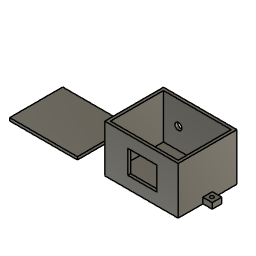
Box and lid v1 (Autodesk Fusion 360 design; units mm, degrees)
Autodesk Fusion 360 part; units mm, degrees
sketch "Sketch4" plane through (0, 0, 0) normal (0, 0, 1) x (1, 0, 0)
  line L0 (38.75, -31) -> (-38.75, -31)
  line L1 (-38.75, -31) -> (-38.75, 31)
  line L2 (-38.75, 31) -> (38.75, 31)
  line L3 (38.75, 31) -> (38.75, -31)
  line L4 (38.75, -31) -> (-38.75, 31) construction
  line L5 (-38.75, -31) -> (38.75, 31) construction
  dimension "d14" = 77.5
  dimension "d15" = 62
  constraint horizontal L0
  constraint perpendicular L0 L1
  constraint parallel L0 L2
  constraint parallel L1 L3
  constraint coincident L4 origin
  constraint coincident L5 origin
  measures "d14" distance of L1 L3
  measures "d15" distance of L0 L2
extrude "Extrude4" add sketch "Sketch4" along normal blind 50 makes body 1
sketch "Sketch5" plane through (0, 0, 50) normal (0, 0, 1) x (-1, 0, 0)
  line L0 (-38.75, -31) -> (38.75, -31)
  line L1 (38.75, -31) -> (38.75, 31)
  line L2 (38.75, 31) -> (-38.75, 31)
  line L3 (-38.75, 31) -> (-38.75, -31)
  line L4 (-35.75, 28) -> (35.75, 28)
  line L5 (35.75, 28) -> (35.75, -28)
  line L6 (35.75, -28) -> (-35.75, -28)
  line L7 (-35.75, -28) -> (-35.75, 28)
  line L8 (-35.75, 28) -> (35.75, -28) construction
  line L9 (35.75, 28) -> (-35.75, -28) construction
  dimension "d18" = 71.5
  dimension "d19" = 56
  constraint horizontal L4
  constraint perpendicular L4 L5
  constraint parallel L4 L6
  constraint parallel L5 L7
  constraint coincident L8 origin
  constraint coincident L9 origin
  measures "d18" distance of L5 L7
  measures "d19" distance of L4 L6
extrude "Extrude5" cut sketch "Sketch5" against normal blind 47 contours L4 L5 L6 L7 bodies 1
sketch "Sketch6" plane through (0, -31, 0) normal (0, -1, 0) x (1, 0, 0)
  line L0 (-38.75, 0) -> (38.75, 0)
  line L1 (38.75, 0) -> (38.75, 50)
  line L2 (38.75, 50) -> (-38.75, 50)
  line L3 (-38.75, 50) -> (-38.75, 0)
  line L4 (16.143, 12.6054) -> (-14.457, 12.6054)
  line L5 (-14.457, 12.6054) -> (-14.457, 37.3554)
  line L6 (-14.457, 37.3554) -> (16.143, 37.3554)
  line L7 (16.143, 37.3554) -> (16.143, 12.6054)
  line L8 (16.143, 12.6054) -> (-14.457, 37.3554) construction
  line L9 (-14.457, 12.6054) -> (16.143, 37.3554) construction
  point P0 (0.843, 24.9804)
  dimension "d22" = 30.6
  dimension "d23" = 24.75
  constraint horizontal L4
  constraint perpendicular L4 L5
  constraint parallel L4 L6
  constraint parallel L5 L7
  constraint coincident L8 P0
  constraint coincident L9 P0
  measures "d22" distance of L5 L7
  measures "d23" distance of L4 L6
extrude "Extrude6" cut sketch "Sketch6" against normal blind 5 contours L4 L5 L6 L7 bodies 1
sketch "Sketch7" plane through (0, 31, 0) normal (0, 1, 0) x (-1, 0, 0)
  line L0 (-38.75, 0) -> (38.75, 0)
  line L1 (38.75, 0) -> (38.75, 50)
  line L2 (38.75, 50) -> (-38.75, 50)
  line L3 (-38.75, 50) -> (-38.75, 0)
  line L4 (0, 60) -> (0, -15)
  circle A0 centre (-20, 25) radius 3.675
  circle A1 centre (20, 25) radius 3.675
  dimension "d26" = 7.35
  dimension "d27" = 7.35
  constraint perpendicular L0 L4
  measures "d26" diameter of A0
  measures "d27" diameter of A1
extrude "Extrude7" cut sketch "Sketch7" against normal blind 5 contours A0 bodies 1
extrude "Extrude8" cut sketch "Sketch7" against normal blind 5 contours A1 bodies 1
sketch "Sketch8" plane through (0, 0, 3) normal (0, 0, 1) x (-1, 0, 0)
  line L0 (-35.75, -28) -> (35.75, -28)
  line L1 (35.75, -28) -> (35.75, 28)
  line L2 (35.75, 28) -> (-35.75, 28)
  line L3 (-35.75, 28) -> (-35.75, -28)
  line L4 (49, -5) -> (39, -5)
  line L5 (39, -5) -> (39, 5)
  line L6 (39, 5) -> (49, 5)
  line L7 (49, 5) -> (49, -5)
  dimension "d32" = 10
  dimension "d33" = 10
  constraint horizontal L4
  constraint vertical L5
  constraint horizontal L6
  constraint vertical L7
  measures "d32" distance of L5 L7
  measures "d33" distance of L4 L6
extrude "Extrude9" add sketch "Sketch8" along normal blind 6 separate body contours L4 L5 L6 L7 makes body 2
move_body "Move1" bodies 2 to x (1, 0, 0) y (0, 1, 0) z (0, 0, 1) at (0, 0, -3)
sketch "Sketch9" plane through (0, 0, 3) normal (0, 0, 1) x (1, 0, 0)
move_body "Move2" bodies 2 to x (1, 0, 0) y (0, 1, 0) z (0, 0, 1) at (0.2552, 0.0123, 0.0295)
copy_body "CopyPasteBodies1" bodies 2 makes body 3
move_body "Move3" bodies 3 to x (1, 0, 0) y (0, -1, 0) z (0, 0, -1) at (87.4885, 0.0371, 6.207)
sketch "Sketch10" plane through (0, 0, 6.0295) normal (0, 0, 1) x (-1, 0, 0)
  line L0 (48.7448, 4.9877) -> (38.7448, 4.9877)
  line L1 (38.7448, 4.9877) -> (38.7448, -5.0123)
  line L2 (38.7448, -5.0123) -> (48.7448, -5.0123)
  line L3 (48.7448, -5.0123) -> (48.7448, 4.9877)
  circle A0 centre (43.5, 0) radius 1.825
  circle A1 centre (43.5, 0) radius 1.825
  point P0 (-43.5043, -0.185)
  point P1 (43.5, 0)
  dimension "d36" = 3.65
  dimension "d37" = 3.65
  constraint coincident P1 A0.centre
  measures "d36" diameter of A0
  measures "d37" diameter of A1
extrude "Extrude10" cut sketch "Sketch10" against normal blind 6 contours A0 A1 bodies 2
sketch "Sketch11" plane through (0, 0, 6.1775) normal (0, 0, 1) x (-1, 0, 0)
  line L0 (-48.7437, -5.0248) -> (-38.7437, -5.0248)
  line L1 (-38.7437, -5.0248) -> (-38.7437, 4.9752)
  line L2 (-38.7437, 4.9752) -> (-48.7437, 4.9752)
  line L3 (-48.7437, 4.9752) -> (-48.7437, -5.0248)
  circle A0 centre (-43.4472, -0.0093) radius 1.825
  dimension "d40" = 3.65
  measures "d40" diameter of A0
extrude "Extrude11" cut sketch "Sketch11" against normal blind 6 contours A0 bodies 3
combine "Combine1" operation add target body 2 tool bodies 1 3
sketch "Sketch13" plane through (0, 0, 50) normal (0, 0, 1) x (-1, 0, 0)
  line L0 (35.75, 28) -> (35.75, -28)
  line L1 (35.75, -28) -> (-35.75, -28)
  line L2 (-35.75, -28) -> (-35.75, 28)
  line L3 (-35.75, 28) -> (35.75, 28)
  line L4 (-38.75, -31) -> (38.75, -31)
  line L5 (38.75, -31) -> (38.75, 31)
  line L6 (38.75, 31) -> (-38.75, 31)
  line L7 (-38.75, 31) -> (-38.75, -31)
  line L8 (119.1983, 10) -> (47.6983, 10)
  line L9 (47.6983, 10) -> (47.6983, 66)
  line L10 (47.6983, 66) -> (119.1983, 66)
  line L11 (119.1983, 66) -> (119.1983, 10)
  dimension "d43" = 56
  dimension "d44" = 71.5
  constraint horizontal L8
  constraint vertical L9
  constraint horizontal L10
  constraint vertical L11
  measures "d43" distance of L8 L10
  measures "d44" distance of L9 L11
extrude "Extrude12" add sketch "Sketch13" along normal blind 3 separate body contours L8 L9 L10 L11 makes body 4
move_body "Move4" bodies 4 to x (1, 0, 0) y (0, 1, 0) z (0, 0, 1) at (0, 0, -50)
move_body "Move5" bodies 4 to x (1, 0, 0) y (0, 1, 0) z (0, 0, 1) at (-20, 35, 0)
extrude "Extrude1" [rolled back] along distance 50 taper angle 0
sketch "Sketch2" plane through (0, 0, 50) normal (0, 0, 1) x (-1, 0, 0)
  line L0 (22.5, 37) -> (-55, 37)
  line L1 (-55, 37) -> (-55, -25)
  line L2 (-55, -25) -> (22.5, -25)
  line L3 (22.5, -25) -> (22.5, 37)
  line L4 (-51.3638, 33.3638) -> (-51.3638, -21.3638)
  line L5 (-51.3638, -21.3638) -> (18.8638, -21.3638)
  line L6 (18.8638, -21.3638) -> (18.8638, 33.3638)
  line L7 (18.8638, 33.3638) -> (-51.3638, 33.3638)
  dimension "d7" = -3.6362
extrude "Extrude2" [rolled back] along distance -30 taper angle 0
extrude "Extrude3" [rolled back] along distance -47 taper angle 0
sketch "Sketch3" plane through (0, -37, 0) normal (0, -1, 0) x (1, 0, 0)
  line L0 (-22.5, 0) -> (55, 0)
  line L1 (55, 0) -> (55, 50)
  line L2 (55, 50) -> (-22.5, 50)
  line L3 (-22.5, 50) -> (-22.5, 0)
  line L4 (1.8537, 36.4577) -> (32.4537, 36.4577)
  line L5 (32.4537, 36.4577) -> (32.4537, 11.7577)
  line L6 (32.4537, 11.7577) -> (1.8537, 11.7577)
  line L7 (1.8537, 11.7577) -> (1.8537, 36.4577)
  dimension "d12" = 24.7
  dimension "d13" = 30.6
  constraint horizontal L4
  constraint vertical L5
  constraint horizontal L6
  constraint vertical L7
  measures "d12" distance of L4 L6
  measures "d13" distance of L5 L7
